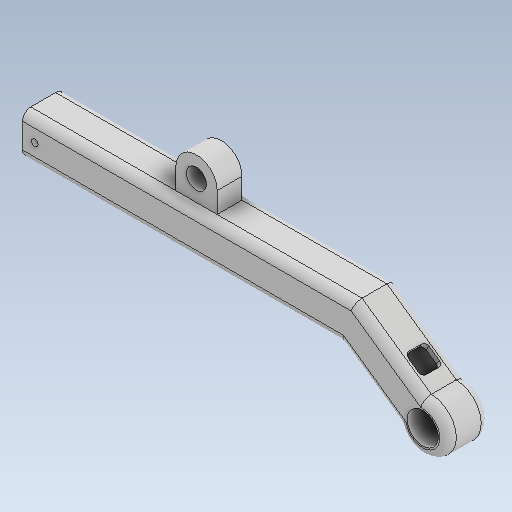
# Autodesk Inventor part: Fahrwerk_rocker_hinten
Saved by Autodesk Inventor 2021 (Build 250183000, 183)
## iProperties
Created: 2020-12-28
Part Number: Fahrwerk_rocker_hinten
Material: Generisch
Document SubType Name: Modeling
Designer: laure
Density: 1 g/cm^3
Appearance: Vorgabe
Author: laure
Autodesk Inventor part; units mm, degrees
ref_plane "YZ Plane" through (0, 0, 0) normal (1, 0, 0) x (0, 1, 0)
ref_plane "XZ Plane" through (0, 0, 0) normal (0, 1, 0) x (-1, 0, 0)
sketch "Skizze1" plane through (0, 0, 0) normal (0, 0, 1) x (1, 0, 0)
  line L0 (-110, 10) -> (50, 10)
  line L1 (43.694024, -10) -> (-110, -10)
  line L2 (-151.829825, 0) -> (140.978947, 0)
  line L3 (87.677594, -40.797627) -> (43.694024, -10)
  line L4 (50, 10) -> (99.149123, -24.414586)
  line L5 (99.149123, -24.414586) -> (87.677594, -40.797627)
  line L6 (0, -50.957152) -> (0, 20.159525)
  line L7 (-110, 10) -> (-110, -10)
  point P0 (0, 0)
  dimension "d5" = 20
  dimension "d56" = 0
  dimension "d57" = 0
  dimension "d58" = 60
  dimension "d138" = 160
  constraints: 12 end point, 2 parallel, 1 horizontal, 1 perpendicular, 1 other
  measures "d5" distance between parallel lines of L4 L3
  measures "d56" distance from line of L0 L4.start
  measures "d57" distance of L0.end L4.start
  measures "d58" distance from line of L4.start L5
  measures "d138" distance from line of L7 L0.end
sketch "Skizze4" plane through (0, 0, 0) normal (0, 0, 1) x (1, 0, 0)
  line L0 (-40, 10) -> (-20, 10)
  line L1 (-20, 10) -> (-20, 20)
  line L2 (-30, 30) -> (-30, 30)
  line L3 (-40, 20) -> (-40, 10)
  circle A0 centre (-30, 20) radius 4.875
  arc A1 (-30, 30) -> (-40, 20) centre (-30, 20) ccw
  arc A2 (-20, 20) -> (-30, 30) centre (-30, 20) ccw
  line L4 (-50.485282, 0) -> (8.414214, 0)
  line L5 (0, -6.414214) -> (0, 38.485282)
  point P0 (0, 0)
  point P1 (-30, 30)
  dimension "d74" = 20
  dimension "d75" = 20
  dimension "d76" = 9.75
  dimension "d77" = 10
  dimension "d78" = 10
  dimension "d115" = 10
  dimension "d116" = 10
  dimension "d139" = 30
  constraints: 8 end point, 4 point on circle, 4 tangent, 3 centre point, 2 parallel, 1 concentric, 1 horizontal, 1 perpendicular
  measures "d74" distance between parallel lines of L1 L3
  measures "d75" distance between parallel lines of L0 L2
  measures "d76" diameter of A0
  measures "d77" distance from line of A0.centre L0
  measures "d78" radius of A1
  measures "d115" distance from line of L3 A0.centre
  measures "d116" distance between parallel lines of L0 L4
  measures "d139" distance from line of L5 A0.centre
extrude "Extrusion1" add sketch "Skizze1" against normal mid plane 20
sketch "Skizze7" plane through (0, 0, -10) normal (0, 0, -1) x (-1, 0, 0)
  circle A0 centre (-83.3, -25.7) radius 7.5
  line L0 (-83.3, -25.7) -> (-83.3, -18.2)
  circle A1 centre (-83.3, -25.7) radius 12.25
  circle A2 centre (-83.3, -25.7) radius 8.937752
  point P0 (0, 0)
  dimension "d104" = 24.5
  constraints: 2 centre point, 2 coincident, 2 end point, 1 vertical, 1 vertical alignment, 1 other
  measures "d104" diameter of A1
extrude "Extrusion6" add sketch "Skizze7" against normal blind 20 contours A1
sketch "Skizze8" plane through (0, 0, -10) normal (0, 0, -1) x (-1, 0, 0)
  circle A0 centre (-83.3, -25.7) radius 7.5 projected
  circle A1 centre (-83.3, -25.7) radius 7.5
  point P0 (0, 0)
  constraints: 2 coincident, 1 centre point, 1 concentric
extrude "Extrusion7" cut sketch "Skizze8" against normal blind 20
sketch "Skizze10" plane through (0, 0, -10) normal (0, 0, -1) x (-1, 0, 0)
  circle A0 centre (-83.3, -25.7) radius 7.5
  circle A1 centre (-83.3, -25.7) radius 12.245558
  line L0 (-87.677594, -40.797627) -> (-93.141776, -32.993967)
  arc A2 (-83.492225, -13.451508) -> (-94.744073, -21.330137) centre (-83.3, -25.7) ccw
  arc A3 (-83.605326, -37.946194) -> (-71.687914, -29.601533) centre (-83.3, -25.7) ccw
  line L1 (-99.149123, -24.414586) -> (-93.520172, -32.453561)
  line L2 (-94.744073, -21.330137) -> (-99.149123, -24.414586)
  line L3 (-94.744073, -21.330137) -> (-99.149123, -24.414586)
  line L4 (-87.677594, -40.797627) -> (-99.149123, -24.414586)
  line L5 (-87.677594, -40.797627) -> (-83.605326, -37.946194)
  arc A4 (-94.744073, -21.330137) -> (-83.605326, -37.946194) centre (-83.3, -25.7) ccw
  point P0 (0, 0)
  point P1 (-93.141776, -32.993967)
  constraints: 6 end point, 3 perpendicular, 3 point on circle, 2 centre point, 1 coincident, 1 tangent
extrude "Extrusion9" cut sketch "Skizze10" against normal blind 20 contours A4 L5 L0 | L1 L2 A4
shell "Wandung1" thickness 2.6 removed faces 1 at (-110, -3.333333, -3.333333)
ref_plane "Arbeitsebene1" through (83.492225, -13.451508, 6) normal (0.5735764, 0.819152, 0) x (0.819152, -0.5735764, 0)
sketch "Skizze11" plane through (83.492225, -13.451508, 6) normal (0.5735764, 0.819152, 0) x (0.819152, -0.5735764, 0)
  line L0 (-16.810932, 1) -> (-6.810932, 1)
  line L1 (-6.810932, 1) -> (-6.810932, 11)
  line L2 (-6.810932, 11) -> (-16.810932, 11)
  line L3 (-16.810932, 11) -> (-16.810932, 1)
  line L4 (0, 0) -> (-40.886457, 0)
  point P0 (-76.108295, 6)
  dimension "d123" = 10
  dimension "d124" = 10
  dimension "d125" = 1
  constraints: 8 end point, 2 parallel, 1 horizontal, 1 perpendicular
  measures "d123" distance of L2.end L1.end
  measures "d124" distance of L1.end L0.end
  measures "d125" distance between parallel lines of L4 L0
extrude "Extrusion10" cut sketch "Skizze11" against normal blind 4
extrude "Extrusion11" add sketch "Skizze4" against normal mid plane 12
fillet "Rundung5" radius 4 18 edges at (-30, 10, 10) (-33.153, -10, 10) (-30, 10, -10) (-33.153, -10, -10) (57.691, -19.8008, -10) (66.7461, -1.7258, -10) (66.7461, -1.7258, 10) (57.691, -19.8008, 10) (90.3263, -15.6654, 10) (95.4765, -27.0398, 10) (76.2737, -35.7346, 10) (93.3346, -32.7263, 10) (88.9455, -36.5715, 10) (90.3263, -15.6654, -10) (95.4765, -27.0398, -10) (76.2737, -35.7346, -10) (93.3346, -32.7263, -10) (88.9455, -36.5715, -10)
fillet "Rundung6" radius 2 4 edges at (68.9759, -4.8741, 5) (68.9759, -4.8741, -5) (77.1674, -10.6098, 5) (77.1674, -10.6098, -5)
sketch "Skizze12" plane through (0, 0, 10) normal (0, 0, 1) x (1, 0, 0)
  circle A0 centre (-104, 0) radius 1.6
  line L0 (-110, 6) -> (48.738805, 6)
  line L1 (-110, 6) -> (-110, -6)
  point P0 (0, 0)
  dimension "d133" = 3.2
  dimension "d134" = 6
  dimension "d135" = 6
  constraints: 1 centre point
  measures "d133" diameter of A0
  measures "d134" distance from line of L0 A0.centre
  measures "d135" distance from line of L1 A0.centre
extrude "Extrusion12" cut sketch "Skizze12" against normal up to surface (20 mm away)
